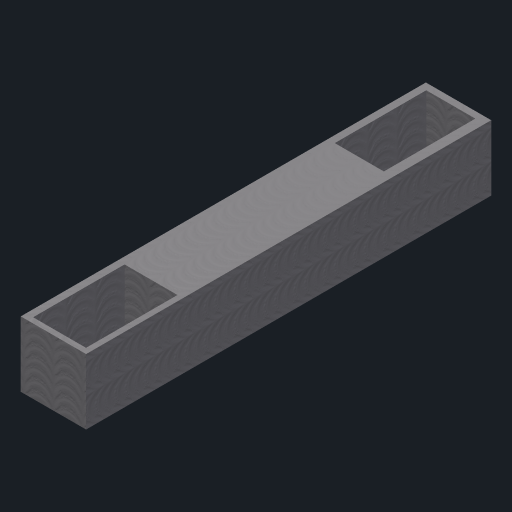
# Autodesk Inventor part: TUBO
Saved by Autodesk Inventor 2024.3 (Build 283343000, 343)
## iProperties
Created: 2024-08-24
Part Number: TUBO
Material: Steel, Mild, Welded
Document SubType Name: Modeling
Designer: Niler
Density: 7.85 g/cm^3
Appearance: Weld - Steel Mild
Author: Niler
Autodesk Inventor part; units mm, degrees
ref_plane "YZ Plane" through (0, 0, 0) normal (1, 0, 0) x (0, 1, 0)
ref_plane "XZ Plane" through (0, 0, 0) normal (0, 1, 0) x (-1, 0, 0)
ref_plane "XY Plane" through (0, 0, 0) normal (0, 0, 1) x (1, 0, 0)
sketch "Sketch1" plane through (0, 0, 0) normal (0, 0, 1) x (1, 0, 0)
  line L0 (-50, -50) -> (50, -50)
  line L1 (50, -50) -> (50, 50)
  line L2 (50, 50) -> (-50, 50)
  line L3 (-50, 50) -> (-50, -50)
  line L4 (-50, -50) -> (50, 50) construction
  line L5 (50, -50) -> (-50, 50) construction
  point P0 (0, 0)
  dimension "d0" = 100
  dimension "d1" = 100
  constraints: 12 end point, 2 midpoint, 2 parallel, 1 horizontal, 1 perpendicular
  measures "d0" distance of L2.end L1.end
  measures "d1" distance of L1.end L0.end
extrude "Extrusion1" add sketch "Sketch1" along normal blind 620
sketch "Sketch2" plane through (-50, -50, 0) normal (0, -1, 0) x (1, 0, 0)
  line L0 (0, 0) -> (100, 0) projected
  line L1 (100, 0) -> (100, 620) projected
  line L2 (0, 620) -> (100, 620) projected
  line L3 (0, 0) -> (0, 620) projected
  line L4 (91.6066, 611.7499) -> (10.6457, 611.7499)
  line L5 (10.6457, 611.7499) -> (10.6457, 471.7499)
  line L6 (10.6457, 471.7499) -> (91.6066, 471.7499)
  line L7 (91.6066, 471.7499) -> (91.6066, 611.7499)
  line L8 (85.7716, 150.054) -> (10.6457, 150.054)
  line L9 (10.6457, 150.054) -> (10.6457, 10.054)
  line L10 (10.6457, 10.054) -> (85.7716, 10.054)
  line L11 (85.7716, 10.054) -> (85.7716, 150.054)
  point P0 (50, 0)
  dimension "d4" = 140
  dimension "d5" = 140
  constraints: 16 end point, 4 parallel, 2 horizontal, 2 perpendicular, 1 point on line
  measures "d4" distance of L5.end L4.end
  measures "d5" distance of L9.end L8.end
extrude "Extrusion2" cut sketch "Sketch2" against normal blind 620 contours L7 L6 L5 L4 | L11 L10 L9 L8
body "Solid1"
